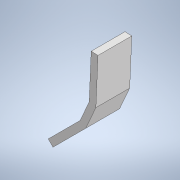
# Autodesk Inventor part: leg_holder_1
Saved by Autodesk Inventor 2020 (Build 240168000, 168)
## iProperties
Created: 2020-12-10
Part Number: leg_holder_1
Material: Generic
Document SubType Name: Modeling
Designer: Shuang Peng
Density: 1 g/cm^3
Appearance: Default
Author: Shuang Peng
Autodesk Inventor part; units mm, degrees
ref_plane "YZ Plane" through (0, 0, 0) normal (1, 0, 0) x (0, 1, 0)
ref_plane "XZ Plane" through (0, 0, 0) normal (0, 1, 0) x (-1, 0, 0)
ref_plane "XY Plane" through (0, 0, 0) normal (0, 0, 1) x (1, 0, 0)
sketch "Sketch1" plane through (0, 0, 0) normal (0, 0, 1) x (1, 0, 0)
  line L0 (32.3537, 16.5891) -> (29.3568, 16.7256) projected
  line L1 (32.3537, 16.5891) -> (32.8543, 27.5777) projected
  line L2 (29.8574, 27.7142) -> (32.8543, 27.5777) projected
  line L3 (29.8574, 27.7142) -> (29.3568, 16.7256) projected
  circle A0 centre (3.6798, 7.8202) radius 1 projected
  circle A1 centre (-7.8202, -3.6798) radius 1 projected
  arc A2 (-1.5944, -1.6537) -> (-1.7076, -1.1208) centre (-2.0611, -1.4744) ccw projected
  line L4 (-1.7076, -1.1208) -> (-2.7902, -0.0382) projected
  arc A3 (-2.7902, 0.6689) -> (-2.7902, -0.0382) centre (-2.4366, 0.3153) ccw projected
  line L5 (-2.7902, 0.6689) -> (-0.6689, 2.7902) projected
  arc A4 (0.0382, 2.7902) -> (-0.6689, 2.7902) centre (-0.3153, 2.4366) ccw projected
  line L6 (0.0382, 2.7902) -> (1.1208, 1.7076) projected
  arc A5 (1.1208, 1.7076) -> (1.6537, 1.5944) centre (1.4744, 2.0611) ccw projected
  arc A6 (-1.5944, -1.6537) -> (1.6537, 1.5944) centre (3.6798, -3.6798) ccw projected
  circle A7 centre (3.6798, -15.1798) radius 1 projected
  circle A8 centre (15.1798, -3.6798) radius 1 projected
  circle A9 centre (-10.1088, 10.1088) radius 3.075 projected
  line L7 (13.8898, -7.9883) -> (15.3389, -10.0747) projected
  arc A10 (15.1676, -11.991) -> (15.3389, -10.0747) centre (14.107, -10.9304) ccw projected
  line L8 (15.1676, -11.991) -> (11.991, -15.1676) projected
  arc A11 (10.0747, -15.3389) -> (11.991, -15.1676) centre (10.9304, -14.107) ccw projected
  line L9 (10.0747, -15.3389) -> (7.9883, -13.8898) projected
  arc A12 (7.7833, -11.5972) -> (7.9883, -13.8898) centre (8.844, -12.6578) ccw projected
  line L10 (7.7833, -11.5972) -> (11.5972, -7.7833) projected
  arc A13 (13.8898, -7.9883) -> (11.5972, -7.7833) centre (12.6578, -8.844) ccw projected
  line L11 (-7.8202, -5.6798) -> (-6.7452, -5.6798) projected
  arc A14 (-5.3309, -6.2656) -> (-6.7452, -5.6798) centre (-6.7452, -7.6798) ccw projected
  line L12 (-5.3309, -6.2656) -> (1.094, -12.6906) projected
  arc A15 (1.6798, -14.1048) -> (1.094, -12.6906) centre (-0.3202, -14.1048) ccw projected
  line L13 (1.6798, -14.1048) -> (1.6798, -15.1798) projected
  arc A16 (1.6798, -15.1798) -> (2.7432, -16.9469) centre (3.6798, -15.1798) ccw projected
  line L14 (2.7432, -16.9469) -> (10.3973, -21.0039) projected
  line L15 (10.3973, -21.0039) -> (21.0039, -10.3973) projected
  line L16 (21.0039, -10.3973) -> (16.9469, -2.7432) projected
  arc A17 (16.9469, -2.7432) -> (15.1798, -1.6798) centre (15.1798, -3.6798) ccw projected
  line L17 (15.1798, -1.6798) -> (14.1048, -1.6798) projected
  arc A18 (12.6906, -1.094) -> (14.1048, -1.6798) centre (14.1048, 0.3202) ccw projected
  line L18 (12.6906, -1.094) -> (6.2656, 5.3309) projected
  arc A19 (5.6798, 6.7452) -> (6.2656, 5.3309) centre (7.6798, 6.7452) ccw projected
  line L19 (5.6798, 6.7452) -> (5.6798, 7.8202) projected
  arc A20 (5.6798, 7.8202) -> (4.5964, 9.5978) centre (3.6798, 7.8202) ccw projected
  line L20 (4.5964, 9.5978) -> (-10.1088, 17.1798) projected
  arc A21 (-12.2301, 17.1798) -> (-10.1088, 17.1798) centre (-11.1694, 18.2405) ccw projected
  line L21 (-12.2301, 17.1798) -> (-13.6443, 18.594) projected
  line L22 (-18.594, 13.6443) -> (-13.6443, 18.594) projected
  line L23 (-17.1798, 12.2301) -> (-18.594, 13.6443) projected
  arc A22 (-17.1798, 10.1088) -> (-17.1798, 12.2301) centre (-18.2405, 11.1694) ccw projected
  line L24 (-17.1798, 10.1088) -> (-9.5978, -4.5964) projected
  arc A23 (-9.5978, -4.5964) -> (-7.8202, -5.6798) centre (-7.8202, -3.6798) ccw projected
  line L25 (10.3973, -21.0039) -> (24.5395, -6.8618)
  line L26 (24.5395, -6.8618) -> (28.5756, 2.2875)
  line L27 (28.5756, 2.2875) -> (29.4857, 22.2668)
  line L28 (10.3973, -21.0039) -> (29.4857, 22.2668)
  line L29 (10.3973, -21.0039) -> (12.5187, -23.1253)
  line L30 (12.5187, -23.1253) -> (27.0577, -8.5862)
  line L31 (27.0577, -8.5862) -> (31.5469, 1.5902)
  line L32 (31.5469, 1.5902) -> (32.4826, 22.1303)
  line L33 (32.4826, 22.1303) -> (29.4857, 22.2668)
  point P0 (0, 0)
  dimension "d0" = 20
  dimension "d1" = 10
  dimension "d2" = 20
  dimension "d3" = 3
  dimension "d4" = 3
  dimension "d5" = 3
  constraints: 18 end point, 4 parallel, 3 perpendicular, 1 collinear
  measures "d0" distance of L14.end L25.end
  measures "d1" distance of L25.end L26.end
  measures "d2" distance of L26.end L27.end
  measures "d3" distance of L14.end L29.end
  measures "d4" distance of L27.end L32.end
  measures "d5" distance between parallel lines of L26 L31
extrude "Extrusion1" add sketch "Sketch1" against normal blind 15 contours L32 L31 L30 L29 L15 L25 L26 L27 L33 L3 L0 | L0 L3 L33 L32
ref_plane "Work Plane1" through (-35.8496, 25.243, 0) normal (-0.4036, -0.9149, 0) x (0, 0, 1)
body "Solid1"
